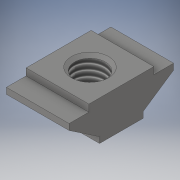
# Autodesk Inventor part: Robotunits TIN_4508
Saved by Autodesk Inventor 2019 (Build 230136000, 136)
## iProperties
Created: 2023-08-22
Part Number: Robotunits TIN_4508
Material: Generic
Catalog Web Link: www.cadenas.de
Description: TIN 450_-Drop-in nut
Vendor: ROBOTUNITS
Document SubType Name: Modeling
Designer: psAdmin
Manufacturer: ROBOTUNITS
Mass: 10 g
Surface Area: 11.1246 cm^2
Volume: 1.48782 cm^3
Density: 7.85 g/cm^3
Appearance: PSOLRGB-128-128-128
Category: PARTsolutions
Company: ROBOTUNITS
Title: Robotunits TIN_4508
Author: Cadenas PARTsolutions
Comments: Drop-in nut
PSOL_IDENT_0: {$CADENAS_DATA/23d-libs/robotunits/pool_bauteile/tin_450.prj},180 {VTYP=3D},{NB=Robotunits TIN_4508}
PSOL_IDENT_1: ,{LINA=Robotunits TIN_4508},{NN=TIN 450_},{DATE=03.03.2023 08:37:04},{GEOMDATE=03.03.2023 08:35:36},
PSOL_IDENT_2: {VERSION=},{LINEID=50},{WBVAR=},{WBNUMERIC=}  {NB=Robotunits TIN_4508},{LINA=Robotunits TIN_4508},{K
PSOL_IDENT_3: T=DUMMY},{ARTIKEL=TIN_4508},{M=M8},{NDM=8.000},{KDM=6.647},{GEW=0.010},{VERS=4508},{ROB=TIN4508},{RO
PSOL_IDENT_4: BX=http://www.robotunits.com/$CADENAS_LANGUAGE./Webshop/Verbindungstechnik/shopitem/einschwenkmutter
PSOL_IDENT_5: /193/},{ZOLL=73181900}
NB: Robotunits TIN_4508
NN: TIN 450_
NT: Drop-in nut
NBSYN: Robotunits $ARTIKEL.
LINA: Robotunits TIN_4508
CATALOG: Robotunits
ARTIKEL: TIN_4508
M: M8
GEW: 0.010
ROB: TIN4508
ZOLL: 73181900
SUPPLIER: ROBOTUNITS
ARTICLENO: Robotunits TIN_4508
BOMINFO: Robotunits TIN_4508
CREATOR: CADENAS GmbH
Autodesk Inventor part; units mm, degrees
sketch "Skizze_1" plane through (0, 0, 0) normal (1, 0, 0) x (0, 1, 0)
  line L0 (5.7, 11.25) -> (1.275, 4.7)
  line L1 (1.275, 4.7) -> (0, 4.7)
  line L2 (0, 4.7) -> (0, -4.7)
  line L3 (0, -4.7) -> (1.275, -4.7)
  line L4 (1.275, -4.7) -> (5.7, -11.25)
  line L5 (5.7, -11.25) -> (7, -11.25)
  line L6 (7, -11.25) -> (7, -7)
  line L7 (7, -7) -> (8.5, -7)
  line L8 (8.5, -7) -> (8.5, 7)
  line L9 (8.5, 7) -> (7, 7)
  line L10 (7, 7) -> (7, 11.25)
  line L11 (7, 11.25) -> (5.7, 11.25)
  constraints: 24 end point
extrude "Extrusion1" add sketch "Skizze_1" along normal mid plane 13.5
sketch "Skizze_2" plane through (0, 0, 0) normal (0, 0, 1) x (1, 0, 0)
  line L0 (0, 0) -> (0, 8.5)
  line L1 (0, 8.5) -> (4, 8.5)
  line L2 (4, 8.5) -> (3.3235, 7.8235)
  line L3 (3.3235, 7.8235) -> (3.3235, 0.6765)
  line L4 (3.3235, 0.6765) -> (4, 0)
  line L5 (4, 0) -> (0, 0)
  line L6 (0, 0) -> (0, 8.5)
  constraints: 14 end point
revolve "Revolution1" cut sketch "Skizze_2" angle 360 about axis through (0, 0, 0) along (0, -1, 0)
thread "Thread1" size "M8x1.25" class "6H" standard "ISO Metric profile" full length
ref_plane "TIN_4_XY" through (0, 8.5, 0) normal (0, 1, 0) x (1, 0, 0)
ref_plane "TIN_4_YZ" through (0, 8.5, 0) normal (1, 0, 0) x (0, 0, -1)
ref_plane "TIN_4_ZX" through (0, 8.5, 0) normal (0, 0, -1) x (0, 1, 0)
body "Solid1"
